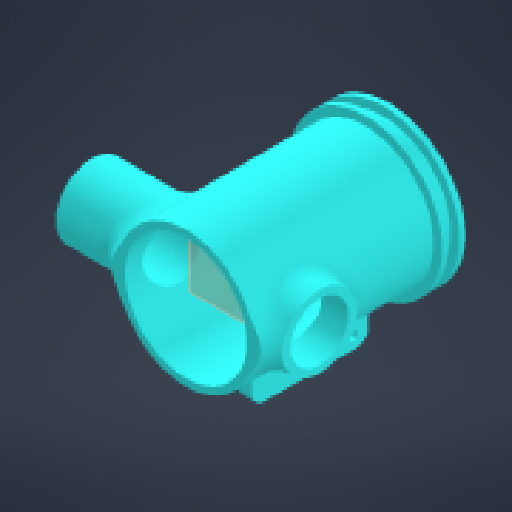
# Autodesk Inventor part: lower_arm
Saved by Autodesk Inventor 2024 (Build 280153000, 153)
## iProperties
Created: 2023-04-15
Part Number: lower_arm
Material: Типовые
Document SubType Name: Modeling
Designer: user
Density: 1 g/cm^3
Appearance: По умолчанию
Author: user
Autodesk Inventor part; units mm, degrees
ref_plane "YZ Plane" through (0, 0, 0) normal (1, 0, 0) x (0, 1, 0)
ref_plane "XZ Plane" through (0, 0, 0) normal (0, 1, 0) x (-1, 0, 0)
ref_plane "XY Plane" through (0, 0, 0) normal (0, 0, 1) x (1, 0, 0)
sketch "Эскиз1" plane through (0, 0, 0) normal (0, 0, 1) x (1, 0, 0)
  circle A0 centre (0, 0) radius 21
  circle A1 centre (0, 0) radius 21 projected
  circle A2 centre (0, 0) radius 23.5
  dimension "d2" = 42
  dimension "d3" = 47
  constraints: 2 centre point, 2 coincident, 1 concentric
  measures "d2" diameter of A0
  measures "d3" diameter of A2
extrude "Выдавливание1" add sketch "Эскиз1" against normal blind 70
ref_plane "РабПлоскость2" through (0, 0, -16) normal (0, 0, 1) x (1, 0, 0)
sketch "Эскиз3" plane through (0, 0, -16) normal (0, 0, 1) x (1, 0, 0)
  line L0 (-19.899749, -12.5) -> (-48.5, -12.5)
  line L1 (-48.5, -12.5) -> (-48.5, 12.5)
  line L2 (-48.5, 12.5) -> (-19.899749, 12.5)
  line L3 (19.899749, -12.5) -> (35.16, -12.5)
  line L4 (35.16, -12.5) -> (35.16, 12.5)
  line L5 (35.16, 12.5) -> (19.899749, 12.5)
  arc A0 (19.899749, -12.5) -> (19.899749, 12.5) centre (0, 0) ccw
  arc A1 (-19.899749, 12.5) -> (-19.899749, -12.5) centre (0, 0) ccw
  circle A2 centre (0, 0) radius 23.5
  line L6 (35.16, 0) -> (23.5, 0)
  line L7 (-23.5, 0) -> (-48.5, 0)
  dimension "d11" = 25
  dimension "d36" = 48.5
  dimension "d37" = 35.16
  constraints: 16 end point, 11 point on circle, 4 point on line, 3 perpendicular, 2 centre point, 2 midpoint, 1 coincident, 1 horizontal, 1 horizontal alignment
  measures "d11" distance of L0.end L1.end
  measures "d36" horizontal distance of point (0, 0) L0.end
  measures "d37" horizontal distance of L3.end point (0, 0)
revolve "Вращение1" add sketch "Эскиз3" angle 360 about axis through (35.16, 0, -16) along (-1, 0, 0) contours L0 L1 L7 A1 | A0 L6 L4 L3
fillet "Сопряжение1" radius 10 6 edges at (21.4934, -9.5017, -24.1221) (21.4932, 9.5022, -24.1214) (21.4934, -9.5017, -7.878) (21.4921, 9.5046, -7.8814) (-23.5, -0.0017, -28.5) (-23.5, 0.0063, -3.5)
sketch "Эскиз4" plane through (35.16, 0, -16) normal (1, 0, 0) x (0, 0, -1)
  circle A0 centre (0, 0) radius 10
  point P0 (-16, 0)
  dimension "d14" = 20
  constraints: 1 centre point
  measures "d14" diameter of A0
extrude "Выдавливание2" cut sketch "Эскиз4" against normal through all
sketch "Эскиз5" plane through (0, 0, -16) normal (0, 0, 1) x (1, 0, 0)
  line L0 (-7, -22.433234) -> (-7, -34.433234)
  line L1 (-7, -34.433234) -> (-2, -34.433234)
  line L2 (-2, -34.433234) -> (-2, -23.414739)
  line L3 (2, -23.414739) -> (2, -34.433234)
  line L4 (2, -34.433234) -> (7, -34.433234)
  line L5 (7, -34.433234) -> (7, -22.433234)
  arc A0 (-7, -22.433234) -> (-2, -23.414739) centre (0, 0) ccw
  arc A1 (2, -23.414739) -> (7, -22.433234) centre (0, 0) ccw
  line L6 (-2, -34.433234) -> (2, -34.433234) construction
  circle A2 centre (0, 0) radius 23.5 construction
  point P0 (0, -34.433234)
  dimension "d17" = 12
  dimension "d18" = 5
  dimension "d19" = 4
  constraints: 14 end point, 6 point on circle, 3 perpendicular, 2 centre point, 2 collinear, 2 point on line, 1 coincident, 1 midpoint, 1 parallel, 1 vertical, 1 vertical alignment
  measures "d17" distance of L0.start L0.end
  measures "d18" distance of L0.end L1.end
  measures "d19" distance of L1.end L3.end
extrude "Выдавливание3" add sketch "Эскиз5" against normal blind 40
sketch "Эскиз6" plane through (7, -34.433234, -16) normal (1, 0, 0) x (0, 0, -1)
  circle A0 centre (35, 4) radius 1.5
  circle A1 centre (27, 4) radius 1.5
  circle A2 centre (19, 4) radius 1.5
  line L0 (40, 12) -> (40, 0) projected
  line L1 (35, 4) -> (27, 4) construction
  line L2 (27, 4) -> (19, 4) construction
  point P0 (-16, 34.433234)
  point P1 (40, 6)
  dimension "d22" = 3
  dimension "d23" = 5
  dimension "d24" = 8
  dimension "d34" = 4
  constraints: 4 end point, 3 centre point, 2 collinear, 2 equal radius, 2 horizontal alignment, 1 horizontal, 1 midpoint
  measures "d22" diameter of A0
  measures "d23" horizontal distance of L0.end L1.start
  measures "d24" distance of L1.start L1.end
  measures "d34" vertical distance of L0.end L1.start
extrude "Выдавливание4" cut sketch "Эскиз6" against normal through all
fillet "Сопряжение2" radius 4 8 edges at (4.5, -34.4332, -56) (-4.5, -34.4332, -56) (4.5, -34.4332, -16) (-4.5, -34.4332, -16) (4.5267, -23.0599, -56) (-4.5267, -23.0599, -56) (-4.5267, -23.0599, -16) (4.5267, -23.0599, -16)
sketch "Эскиз7" plane through (0, 0, 0) normal (0, 0, 1) x (1, 0, 0)
  circle A0 centre (0, 0) radius 21 projected
extrude "Выдавливание5" cut sketch "Эскиз7" against normal blind 94.5
sketch "Эскиз8" plane through (0, 0, 0) normal (1, 0, 0) x (0, 1, 0)
  line L0 (-23.5, -70) -> (23.5, -70) projected
  line L1 (-23.5, -70) -> (-26.5, -70)
  line L2 (-26.5, -70) -> (-26.5, -68)
  line L3 (-26.5, -68) -> (-23.5, -68)
  line L4 (-23.5, -68) -> (-23.5, -70)
  line L5 (-23.5, -64) -> (-26.5, -64)
  line L6 (-26.5, -64) -> (-26.5, -62)
  line L7 (-26.5, -62) -> (-23.5, -62)
  line L8 (-23.5, -62) -> (-23.5, -64)
  line L9 (0, -70) -> (0, 0)
  line L10 (-21, 0) -> (21, 0) projected
  dimension "d30" = 4
  dimension "d31" = 2
  dimension "d32" = 3
  constraints: 18 end point, 4 parallel, 3 perpendicular, 2 horizontal, 2 point on line, 1 collinear, 1 midpoint
  measures "d30" distance of L5.end L2.end
  measures "d31" distance of L5.end L6.end
  measures "d32" distance of L0.start L1.end
revolve "Вращение2" add sketch "Эскиз8" angle 360 about axis through (0, 0, -70) along (0, 0, 1)
fillet "Сопряжение3" radius 4 2 edges at (7, -22.4332, -36) (-7, -22.4332, -36)
